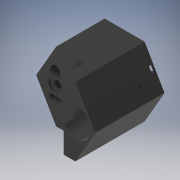
# Autodesk Inventor part: TA02
Saved by Autodesk Inventor 2017 (Build 210142000, 142)
## iProperties
Created: 2018-10-09
Part Number: TA02
Material: ABS Plastic
Document SubType Name: Modeling
Designer: Zach
Density: 1.06 g/cm^3
Appearance: Smooth - Black
Mass: 254.186 g
Surface Area: 673.602 cm^2
Volume: 239.798 cm^3
Author: Zach
Autodesk Inventor part; units mm, degrees
(part 1 of 2)
ref_plane "YZ Plane" through (0, 0, 0) normal (1, 0, 0) x (0, 1, 0)
ref_plane "XZ Plane" through (0, 0, 0) normal (0, 1, 0) x (-1, 0, 0)
ref_plane "XY Plane" through (0, 0, 0) normal (0, 0, 1) x (1, 0, 0)
sketch "Sketch48" plane through (0, 0, 0) normal (0, 0, 1) x (1, 0, 0)
  line L0 (57.5, 0) -> (28.75, -49.7965)
  line L1 (28.75, -49.7965) -> (-28.75, -49.7965)
  line L2 (-28.75, -49.7965) -> (-57.5, 0)
  line L3 (-57.5, 0) -> (-28.75, 49.7965)
  line L4 (-28.75, 49.7965) -> (28.75, 49.7965)
  line L5 (28.75, 49.7965) -> (57.5, 0)
  circle A0 centre (0, 0) radius 7
  circle A1 centre (30, 0) radius 10 construction
  circle A2 centre (-15, 25.9808) radius 5.5
  line L6 (-15, 25.9808) -> (0, 0) construction
  line L7 (0, 0) -> (30, 0) construction
  line L8 (25.6411, -9) -> (34.3589, -9)
  line L9 (25.6411, 9) -> (34.3589, 9)
  arc A3 (25.6411, 9) -> (25.6411, -9) centre (30, 0) ccw
  arc A4 (34.3589, -9) -> (34.3589, 9) centre (30, 0) ccw
  line L10 (21, 9) -> (39, 9) construction
  line L11 (39, 9) -> (39, -9) construction
  line L12 (39, -9) -> (21, -9) construction
  line L13 (21, -9) -> (21, 9) construction
  circle A5 centre (21, 9) radius 2
  circle A6 centre (21, -9) radius 2
  circle A7 centre (39, -9) radius 2
  circle A8 centre (39, 9) radius 2
  point P0 (30, 9)
  point P1 (39, 0)
  dimension "d220" = 115
  dimension "d221" = 14
  dimension "d222" = 30
  dimension "d224" = 30
  dimension "d225" = 120
  dimension "d227" = 11
  dimension "d228" = 20
  dimension "d229" = 18
  dimension "d232" = 18
  dimension "d233" = 18
  dimension "d234" = 4
  dimension "d235" = 4
  dimension "d236" = 4
  dimension "d237" = 4
  constraints: 28 end point, 9 centre point, 8 point on circle, 6 coincident, 3 horizontal, 3 parallel, 2 concentric, 2 horizontal alignment, 2 midpoint, 2 vertical alignment, 1 perpendicular, 13 other
  measures "d220" distance of L0.start L2.end
  measures "d221" diameter of A0
  measures "d222" distance of L7.end point (0, 0)
  measures "d224" distance of point (0, 0) L6.start
  measures "d225" angle of L6 L7
  measures "d227" diameter of A2
  measures "d228" diameter of A1
  measures "d229" distance between parallel lines of L8 L9
  measures "d232" distance of L11.end L12.end
  measures "d233" distance of L10.end L11.end
  measures "d234" diameter of A5
  measures "d235" diameter of A6
  measures "d236" diameter of A7
  measures "d237" diameter of A8
extrude "Extrusion43" add sketch "Sketch48" along normal blind 120
sketch "Sketch49" plane through (0, 0, 0) normal (0, 0, -1) x (-1, 0, 0)
  arc A0 (-34.3589, 9) -> (-34.3589, -9) centre (-30, 0) ccw projected
  circle A1 centre (-30, 0) radius 16.5
  point P0 (0, 0)
  dimension "d238" = 33
  constraints: 1 centre point, 1 coincident
  measures "d238" diameter of A1
extrude "Extrusion44" cut sketch "Sketch49" against normal blind 115
sketch "Sketch50" plane through (0, 0, 0) normal (0, 0, -1) x (-1, 0, 0)
  arc A0 (-34.3589, 9) -> (-34.3589, -9) centre (-30, 0) ccw projected
  circle A1 centre (-30, 0) radius 20
  point P0 (0, 0)
  dimension "d241" = 40
  constraints: 1 centre point, 1 coincident
  measures "d241" diameter of A1
extrude "Extrusion45" cut sketch "Sketch50" against normal blind 75
sketch "Sketch51" plane through (0, 0, 120) normal (0, 0, 1) x (1, 0, 0)
  circle A0 centre (21, 9) radius 2 projected
  arc A1 (25.6411, 9) -> (25.6411, -9) centre (30, 0) ccw projected
  circle A2 centre (21, 9) radius 4.5
  circle A3 centre (21, -9) radius 4.5
  circle A4 centre (39, -9) radius 4.5
  circle A5 centre (39, 9) radius 4.5
  point P0 (0, 0)
  dimension "d244" = 9
  dimension "d247" = 360
  constraints: 4 centre point, 1 coincident, 9 other
  measures "d244" diameter of A2
extrude "Extrusion46" cut sketch "Sketch51" against normal blind 2 contours A0 | A2 A1 | A1 A2 | A3 A1 | A1 A3 | A4 | A5
sketch "Sketch53" plane through (0, 0, 120) normal (0, 0, 1) x (1, 0, 0)
  circle A0 centre (-15, 25.9808) radius 5.5 projected
  circle A1 centre (-15, 25.9808) radius 10
  point P0 (0, 0)
  dimension "d251" = 20
  constraints: 1 centre point, 1 coincident
  measures "d251" diameter of A1
extrude "Extrusion47" cut sketch "Sketch53" against normal blind 5 contours A0 | A1
sketch "Sketch54" plane through (0, 0, 120) normal (0, 0, 1) x (1, 0, 0)
  circle A0 centre (0, 0) radius 12.7
  dimension "d254" = 25.4
  constraints: 1 centre point, 1 coincident
  measures "d254" diameter of A0
extrude "Extrusion48" cut sketch "Sketch54" against normal blind 3.2
sketch "Sketch55" plane through (0, 0, 120) normal (0, 0, 1) x (1, 0, 0)
  circle A0 centre (0, 0) radius 9.56
  dimension "d257" = 19.12
  constraints: 1 centre point, 1 coincident
  measures "d257" diameter of A0
extrude "Extrusion49" cut sketch "Sketch55" against normal blind 12.7
sketch "Sketch56" plane through (0, 0, 0) normal (0, 0, -1) x (-1, 0, 0)
  line L0 (57.5, 0) -> (28.75, 49.7965) projected
  line L1 (28.75, -49.7965) -> (57.5, 0) projected
  line L2 (-28.75, -49.7965) -> (28.75, -49.7965) projected
  line L3 (-57.5, 0) -> (-28.75, -49.7965) projected
  line L4 (-28.75, 49.7965) -> (-57.5, 0) projected
  line L5 (28.75, 49.7965) -> (-28.75, 49.7965) projected
  line L6 (-24.1312, 41.7965) -> (-48.2624, 0)
  line L7 (-48.2624, 0) -> (-24.1312, -41.7965)
  line L8 (-24.1312, -41.7965) -> (24.1312, -41.7965)
  line L9 (24.1312, -41.7965) -> (48.2624, 0)
  line L10 (48.2624, 0) -> (24.1312, 41.7965)
  line L11 (24.1312, 41.7965) -> (-24.1312, 41.7965)
  point P0 (0, 0)
  dimension "d260" = 8
  constraints: 12 end point, 5 other
  measures "d260" distance between parallel lines of L5 L11
extrude "Extrusion50" cut sketch "Sketch56" against normal blind 15 contours L11 L10 L9 L8 L7 L6
sketch "Sketch57" plane through (0, 0, 15) normal (0, 0, -1) x (-1, 0, 0)
  circle A0 centre (0, 0) radius 9.56 projected
extrude "Extrusion51" cut sketch "Sketch57" against normal blind 10
sketch "Sketch58" plane through (0, 0, 0) normal (0, 0, -1) x (-1, 0, 0)
  circle A0 centre (-25.5, -44.1673) radius 2
  circle A1 centre (25.5, -44.1673) radius 2
  circle A2 centre (51, 0) radius 2
  circle A3 centre (25.5, 44.1673) radius 2
  circle A4 centre (-25.5, 44.1673) radius 2
  circle A5 centre (-51, 0) radius 2
  line L0 (-51, 0) -> (51, 0) construction
  point P0 (0, 0)
  point P1 (0, 0)
  dimension "d268" = 360
  dimension "d331" = 102
  dimension "d332" = 4
  constraints: 6 centre point, 2 end point, 1 coincident, 1 horizontal, 1 midpoint, 13 other
  measures "d331" distance of L0.start L0.end
  measures "d332" diameter of A0
extrude "Extrusion52" cut sketch "Sketch58" against normal blind 50
sketch "Sketch59" plane through (0, 0, 0) normal (0, 0, -1) x (-1, 0, 0)
  line L0 (-24.1312, 41.7965) -> (24.1312, 41.7965) construction
  line L1 (28.75, 49.7965) -> (-28.75, 49.7965) construction
  line L2 (0, 41.7965) -> (0, 49.7965) construction
  circle A0 centre (0, 45.7965) radius 2.5
  circle A1 centre (-39.6609, 22.8982) radius 2.5
  circle A2 centre (-39.6609, -22.8982) radius 2.5
  circle A3 centre (0, -45.7965) radius 2.5
  circle A4 centre (39.6609, -22.8982) radius 2.5
  circle A5 centre (39.6609, 22.8982) radius 2.5
  point P0 (0, 0)
  dimension "d272" = 5
  dimension "d275" = 360
  constraints: 6 centre point, 3 midpoint, 2 end point, 13 other
  measures "d272" diameter of A0
extrude "Extrusion53" cut sketch "Sketch59" against normal blind 35
sketch "Sketch60" plane through (0, 0, 15) normal (0, 0, -1) x (-1, 0, 0)
  circle A0 centre (15, 25.9808) radius 5.5 construction
  line L0 (21.5753, 12.3695) -> (-0.0753, 24.8695)
  line L1 (-0.0753, 24.8695) -> (8.4247, 39.592)
  line L2 (8.4247, 39.592) -> (30.0753, 27.092)
  line L3 (30.0753, 27.092) -> (21.5753, 12.3695)
  line L4 (21.5753, 12.3695) -> (8.4247, 39.592) construction
  line L5 (-0.0753, 24.8695) -> (30.0753, 27.092) construction
  line L6 (0, 0) -> (15, 25.9808) construction
  point P0 (10.75, 18.6195)
  dimension "d279" = 17
  dimension "d280" = 25
  constraints: 14 end point, 3 midpoint, 2 parallel, 1 perpendicular, 1 point on line
  measures "d279" distance of L0.end L1.end
  measures "d280" distance of L1.end L2.end
extrude "Extrusion54" cut sketch "Sketch60" against normal blind 94
sketch "Sketch61" plane through (0, 0, 15) normal (0, 0, -1) x (-1, 0, 0)
  line L0 (-7.5897, -33.1458) -> (24.9103, 23.1458)
  line L1 (24.9103, 23.1458) -> (44.8288, 11.6458)
  line L2 (44.8288, 11.6458) -> (12.3288, -44.6458)
  line L3 (12.3288, -44.6458) -> (-7.5897, -33.1458)
  line L4 (-7.5897, -33.1458) -> (44.8288, 11.6458) construction
  line L5 (24.9103, 23.1458) -> (12.3288, -44.6458) construction
  line L6 (18.6195, -10.75) -> (0, 0)
  line L7 (0, 0) -> (0, 4.3773)
  point P0 (8.6603, -5)
  dimension "d283" = 65
  dimension "d284" = 23
  dimension "d285" = 10
  dimension "d286" = 120
  constraints: 16 end point, 3 midpoint, 2 parallel, 1 perpendicular, 1 point on line, 1 vertical
  measures "d283" distance of L1.end L2.end
  measures "d284" distance of L0.end L1.end
  measures "d285" distance from line of L6.end L0
  measures "d286" angle of L7 L6
extrude "Extrusion55" cut sketch "Sketch61" along normal blind 15 and the other way blind 80
sketch "Sketch63" plane through (0, 0, 0) normal (1, 0, 0) x (0, 1, 0)
  line L0 (-41.7965, 15) -> (-41.7965, 0) projected
  line L1 (-41.7965, 0) -> (-41.7965, 15) projected
  line L2 (8.7965, 15) -> (-41.7965, 15) projected
  line L3 (0, 15) -> (-41.7965, 15) projected
  line L4 (8.7965, 15) -> (0, 15) projected
  line L5 (-13.7965, 15) -> (-38.7965, 15)
  line L6 (-38.7965, 15) -> (-38.7965, 0)
  line L7 (-38.7965, 0) -> (-13.7965, 0)
  line L8 (-13.7965, 0) -> (-13.7965, 15)
  point P0 (0, 0)
  dimension "d300" = 25
  dimension "d301" = 15
  dimension "d302" = 3
  constraints: 8 end point, 2 parallel, 1 horizontal, 1 perpendicular, 1 point on line
  measures "d300" distance of L7.end L6.end
  measures "d301" distance of L6.end L5.end
  measures "d302" distance between parallel lines of L1 L6
extrude "Extrusion57" cut sketch "Sketch63" against normal through all
sketch "Sketch66" plane through (0, 0, 120) normal (0, 0, 1) x (1, 0, 0)
  line L0 (-28.75, 49.7965) -> (28.75, 49.7965) projected
  line L1 (10, 49.7965) -> (10, -49.7965)
  line L2 (-28.75, -49.7965) -> (28.75, -49.7965) projected
  line L3 (10, 49.7965) -> (28.75, 49.7965)
  line L4 (10, -49.7965) -> (28.75, -49.7965)
  line L5 (57.5, 0) -> (28.75, 49.7965) projected
  line L6 (28.75, -49.7965) -> (57.5, 0) projected
  point P0 (0, 0)
  dimension "d317" = 10
  constraints: 6 end point, 2 collinear, 2 point on line, 1 vertical
  measures "d317" distance from line of point (0, 0) L1
extrude "Extrusion58" cut sketch "Sketch66" against normal blind 40
sketch "Sketch67" plane through (0, 0, 120) normal (0, 0, 1) x (1, 0, 0)
  line L0 (10, 7.8288) -> (10, 49.7965) projected
  line L1 (10, 49.7965) -> (-28.75, 49.7965) projected
  line L2 (-28.75, 49.7965) -> (-57.5, 0) projected
  line L3 (-57.5, 0) -> (-28.75, -49.7965) projected
  line L4 (-28.75, -49.7965) -> (10, -49.7965) projected
  line L5 (10, -49.7965) -> (10, -7.8288) projected
  arc A0 (10, 7.8288) -> (10, -7.8288) centre (0, 0) ccw projected
  circle A1 centre (-15, 25.9808) radius 10 projected
  line L6 (10, -7.8288) -> (10, 7.8288) projected
extrude "Extrusion59" cut sketch "Sketch67" against normal blind 70 contours A0 L5 L4 L3 L2 L1 L0 | L6 A0 | A1
sketch "Sketch68" plane through (0, 0, 50) normal (0, 0, 1) x (1, 0, 0)
  circle A0 centre (0, 0) radius 8.0625
  dimension "d337" = 16.125
  constraints: 1 centre point, 1 coincident
  measures "d337" diameter of A0
extrude "Extrusion60" cut sketch "Sketch68" against normal blind 13.7
sketch "Sketch69" plane through (10, -49.7965, 80) normal (-1, 0, 0) x (0, 0, 1)
  line L0 (0, 0) -> (-30, 0) projected
  line L1 (-30, 99.5929) -> (0, 99.5929) projected
  circle A0 centre (-15, 24.8982) radius 10
  line L2 (0, 49.7965) -> (0, 0) projected
  line L3 (0, 49.7965) -> (0, 0)
  line L4 (0, 49.7965) -> (0, 99.5929)
  line L5 (-15, 14.8982) -> (-80, 14.8982)
  line L6 (-80, 14.8982) -> (-80, 34.8982)
  line L7 (-80, 34.8982) -> (-15, 34.8982)
  line L8 (-80, 0) -> (-80, 49.7965) projected
  line L9 (0, 49.7965) -> (-80, 49.7965)
  circle A1 centre (-15, 74.6947) radius 10
  line L10 (-15, 84.6947) -> (-80, 84.6947)
  line L11 (-80, 84.6947) -> (-80, 64.6947)
  line L12 (-80, 64.6947) -> (-15, 64.6947)
  point P0 (-15, 0)
  point P1 (0, 24.8982)
  dimension "d324" = 20
  constraints: 18 end point, 5 symmetric about line, 4 point on circle, 2 centre point, 2 midpoint, 2 perpendicular, 2 tangent, 2 vertical, 2 vertical alignment, 1 horizontal, 1 horizontal alignment, 1 point on line, 1 other
  measures "d324" diameter of A0
extrude "Extrusion61" cut sketch "Sketch69" along normal mid plane 5
sketch "Sketch70" plane through (0, 0, 50) normal (0, 0, 1) x (1, 0, 0)
  circle A0 centre (0, 0) radius 9.56 projected
  line L0 (0, -9.56) -> (30, -9.56)
  line L1 (30, -9.56) -> (30, 9.56)
  line L2 (30, 9.56) -> (0, 9.56)
  arc A1 (0, 9.56) -> (0, -9.56) centre (0, 0) ccw
  arc A2 (37.5759, 18.5096) -> (37.5759, -18.5096) centre (30, 0) ccw projected
  constraints: 6 end point, 4 point on circle, 4 tangent, 1 centre point, 1 horizontal, 1 horizontal alignment, 1 midpoint, 1 perpendicular
extrude "Extrusion62" cut sketch "Sketch70" along normal through all
sketch "Sketch71" plane through (10, 49.7965, 50) normal (-1, 0, 0) x (0, 0, 1)
  line L0 (0, -40.2365) -> (30, -40.2365) projected
  line L1 (30, -40.2365) -> (30, 0) projected
  line L2 (0, 0) -> (30, 0) projected
  line L3 (0, 0) -> (0, -14.8982) projected
  line L4 (0, -14.8982) -> (15, -14.8982) projected
  arc A0 (15, -34.8982) -> (15, -14.8982) centre (15, -24.8982) ccw projected
  line L5 (15, -34.8982) -> (0, -34.8982) projected
  line L6 (0, -34.8982) -> (0, -40.2365) projected
  line L7 (30, -59.3565) -> (0, -59.3565) projected
  line L8 (0, -59.3565) -> (0, -64.6947) projected
  line L9 (0, -64.6947) -> (15, -64.6947) projected
  arc A1 (15, -84.6947) -> (15, -64.6947) centre (15, -74.6947) ccw projected
  line L10 (15, -84.6947) -> (0, -84.6947) projected
  line L11 (0, -84.6947) -> (0, -99.5929) projected
  line L12 (30, -99.5929) -> (0, -99.5929) projected
  line L13 (30, -99.5929) -> (30, -59.3565) projected
  point P0 (-50, -49.7965)
extrude "Extrusion63" cut sketch "Sketch71" against normal blind 1
sketch "Sketch72" plane through (0, 0, 15) normal (0, 0, -1) x (-1, 0, 0)
  line L0 (24.1312, 41.7965) -> (39.8936, 14.4952) projected
  line L1 (8.4247, 39.592) -> (30.0753, 27.092) projected
  line L2 (39.8936, 14.4952) -> (30.0753, 27.092)
  line L3 (30.0753, 27.092) -> (27.0753, 21.8958) projected
  line L4 (27.0753, 21.8958) -> (39.8936, 14.4952) projected
  line L5 (30.0753, 27.092) -> (33.8936, 24.8875)
  line L6 (39.8936, 14.4952) -> (33.8936, 24.8875)
  point P0 (0, 0)
  constraints: 6 end point, 2 collinear, 1 point on line
extrude "Extrusion64" cut sketch "Sketch72" against normal through all
sketch "Sketch73" plane through (0, 0, 15) normal (0, 0, -1) x (-1, 0, 0)
  line L0 (-16.5517, 9.56) -> (-12.4328, 9.56) projected
  arc A0 (-12.4328, 9.56) -> (-12.4328, -9.56) centre (-30, 0) ccw projected
  line L1 (-12.4328, -9.56) -> (-16.5517, -9.56) projected
  arc A1 (-16.5517, 9.56) -> (-16.5517, -9.56) centre (-30, 0) ccw projected
  point P0 (0, 0)
extrude "Extrusion65" cut sketch "Sketch73" along normal through all both and the other way through all
sketch "Sketch74" plane through (0, 0, 50) normal (0, 0, 1) x (1, 0, 0)
  line L0 (7.5, -14.8982) -> (7.5, -34.8982) projected
  line L1 (7.5, -14.8982) -> (4.5, -14.8982)
  line L2 (4.5, -14.8982) -> (4.5, -34.8982)
  line L3 (4.5, -34.8982) -> (7.5, -34.8982)
  line L4 (7.5, -34.8982) -> (7.5, -14.8982)
  point P0 (0, 0)
  point P1 (7.5, -32.9904)
  dimension "d338" = 3
  constraints: 8 end point, 2 parallel, 1 coincident, 1 horizontal, 1 perpendicular
  measures "d338" distance of L2.end L0.end
extrude "Extrusion66" add sketch "Sketch74" against normal blind 35
sketch "Sketch75" plane through (12.5, -49.7965, 80) normal (-1, 0, 0) x (0, 0, 1)
  arc A0 (-15, 64.6947) -> (-15, 84.6947) centre (-15, 74.6947) ccw projected
  arc A1 (-15, 14.8982) -> (-15, 34.8982) centre (-15, 24.8982) ccw projected
  circle A2 centre (-15, 74.6947) radius 4
  circle A3 centre (-15, 24.8982) radius 4
  point P0 (-80, 49.7965)
  dimension "d341" = 8
  dimension "d342" = 8
  constraints: 2 centre point, 2 coincident
  measures "d341" diameter of A2
  measures "d342" diameter of A3
extrude "Extrusion67" add sketch "Sketch75" along normal blind 1
fillet "Fillet1" radius 1 2 edges at (11.5, 24.8982, 61) (11.5, -24.8982, 61)
sketch "Sketch76" plane through (0, 0, 15) normal (0, 0, -1) x (-1, 0, 0)
  line L0 (16.9103, 9.2894) -> (3.9199, 16.7894)
  line L1 (3.9199, 16.7894) -> (6.4199, 21.1195)
  line L2 (19.4103, 13.6195) -> (-0.0753, 24.8695) projected
  line L3 (6.4199, 21.1195) -> (19.4103, 13.6195)
  line L4 (19.4103, 13.6195) -> (16.9103, 9.2894)
  line L5 (19.4103, 13.6195) -> (-0.0753, 24.8695) projected
  line L6 (-4.5, -27.7942) -> (19.4103, 13.6195) projected
  point P0 (0, 0)
  dimension "d346" = 15
  dimension "d349" = 5
  constraints: 8 end point, 3 perpendicular, 2 point on line
  measures "d346" distance of L0.start L0.end
  measures "d349" distance of L0.end L1.end
extrude "Extrusion68" cut sketch "Sketch76" against normal through all
sketch "Sketch78" plane through (0, 0, 80) normal (0, 0, 1) x (1, 0, 0)
  circle A0 centre (21.6375, 42.2965) radius 2.5
  line L0 (11, 49.7965) -> (28.75, 49.7965) projected
  point P0 (0, 0)
  dimension "d352" = 21.6375
  dimension "d353" = 7.5
  dimension "d354" = 5
  constraints: 1 centre point
  measures "d352" horizontal distance of point (0, 0) A0.centre
  measures "d353" distance from line of L0 A0.centre
  measures "d354" diameter of A0
extrude "Extrusion69" cut sketch "Sketch78" against normal through all
sketch "Sketch79" plane through (0, 0, 50) normal (0, 0, 1) x (1, 0, 0)
  circle A0 centre (21.6375, 42.2965) radius 2.5 projected
  circle A1 centre (21.6375, 42.2965) radius 10
  line L0 (21.6375, 32.2965) -> (0, 32.2965)
  line L1 (0, 32.2965) -> (0, 52.2965)
  line L2 (0, 52.2965) -> (21.6375, 52.2965)
  point P0 (0, 0)
  dimension "d357" = 20
  constraints: 6 end point, 2 horizontal, 2 point on circle, 2 tangent, 1 centre point, 1 coincident, 1 vertical, 1 vertical alignment
  measures "d357" diameter of A1
extrude "Extrusion70" cut sketch "Sketch79" along normal blind 20 contours A0 | A1 | A1 L0 L1 L2
sketch "Sketch80" plane through (0, 0, 50) normal (0, 0, 1) x (1, 0, 0)
  line L0 (11, 49.7965) -> (11, 9.56) projected
  arc A0 (23.5117, 43.9509) -> (24.0976, 42.7414) centre (21.6375, 42.2965) ccw projected
  line L1 (-6.4199, 21.1195) -> (0.0753, 24.8695) projected
  line L2 (-6.4199, 21.1195) -> (-3.9199, 16.7894) projected
  line L3 (-3.9199, 16.7894) -> (-16.9103, 9.2894) projected
  line L4 (4.5, -27.7942) -> (-16.9103, 9.2894) projected
  line L5 (4.5, -27.7942) -> (4.5, -34.8982) projected
  line L6 (4.5, -34.8982) -> (4.5545, -34.8982) projected
  line L7 (-12.3288, -44.6458) -> (4.5545, -34.8982) projected
  line L8 (-44.8288, 11.6458) -> (-12.3288, -44.6458) projected
  line L9 (-39.8936, 14.4952) -> (-44.8288, 11.6458) projected
  line L10 (-39.8936, 14.4952) -> (-33.8936, 24.8875) projected
  line L11 (-33.8936, 24.8875) -> (-8.4247, 39.592) projected
  line L12 (0.0753, 24.8695) -> (-8.4247, 39.592) projected
  circle A1 centre (0, 0) radius 8.0625 projected
  circle A2 centre (-51, 0) radius 2 projected
  circle A3 centre (-25.5, -44.1673) radius 2 projected
  circle A4 centre (-25.5, 44.1673) radius 2 projected
  line L13 (7.5, 14.8982) -> (7.5, 34.8982) projected
  line L14 (12.5, 34.8982) -> (7.5, 34.8982) projected
  line L15 (12.5, 32.2965) -> (12.5, 34.8982) projected
  line L16 (12.5, 32.2965) -> (21.6375, 32.2965) projected
  arc A5 (21.6375, 32.2965) -> (30.8902, 46.0895) centre (21.6375, 42.2965) ccw projected
  arc A6 (24.0976, 42.7414) -> (23.5117, 43.9509) centre (25.5, 44.1673) ccw projected
  line L17 (-28.75, 49.7965) -> (28.2519, 49.7965) projected
  line L18 (-57.5, 0) -> (-28.75, 49.7965) projected
  line L19 (-28.75, -49.7965) -> (-57.5, 0) projected
  line L20 (11, -49.7965) -> (-28.75, -49.7965) projected
  line L21 (11, -49.7965) -> (11, -34.8982) projected
  line L22 (11, -34.8982) -> (7.5, -34.8982) projected
  line L23 (7.5, -34.8982) -> (7.5, -14.8982) projected
  line L24 (11, -14.8982) -> (7.5, -14.8982) projected
  line L25 (11, -14.8982) -> (11, -9.56) projected
  line L26 (11, -9.56) -> (12.4328, -9.56) projected
  arc A7 (12.4328, 9.56) -> (12.4328, -9.56) centre (30, 0) ccw projected
  line L27 (12.4328, 9.56) -> (11, 9.56) projected
  line L28 (11, 9.56) -> (11, 14.8982) projected
  line L29 (11, 14.8982) -> (7.5, 14.8982) projected
  line L30 (12.5, 32.2965) -> (11, 32.2965)
  line L31 (11, 32.2965) -> (11, 14.8982)
  line L32 (11, 14.8982) -> (12.5, 14.8982)
  line L33 (12.5, 14.8982) -> (12.5, 32.2965)
  line L34 (29.5487, 48.4131) -> (30.8902, 46.0895) projected
  arc A8 (29.5487, 48.4131) -> (28.2519, 49.7965) centre (21.6375, 42.2965) ccw projected
  constraints: 8 end point, 2 parallel, 1 horizontal, 1 perpendicular
extrude "Extrusion71" add sketch "Sketch80" along normal blind 30 contours L30 L33 L32 L0
sketch "Sketch81" plane through (12.5, -49.7965, 80) normal (-1, 0, 0) x (0, 0, 1)
  line L0 (-10, 82.0929) -> (-8.272, 82.0929) projected
  arc A0 (-8.272, 82.0929) -> (-10, 83.3549) centre (-15, 74.6947) ccw projected
  line L1 (-10, 83.3549) -> (-10, 82.0929) projected
  point P0 (-80, 49.7965)
extrude "Extrusion72" add sketch "Sketch81" along normal blind 1.5
sketch "Sketch82" plane through (0, 0, 50) normal (0, 0, 1) x (1, 0, 0)
  line L0 (7.5, 14.8982) -> (7.5, 34.8982) projected
  line L1 (12.5, 34.8982) -> (7.5, 34.8982) projected
  line L2 (7.5, 34.8982) -> (12.5, 34.8982)
  line L3 (12.5, 34.8982) -> (12.5, 14.8982)
  line L4 (12.5, 14.8982) -> (7.5, 14.8982)
  line L5 (7.5, 14.8982) -> (7.5, 34.8982)
  line L6 (7.5, 14.8982) -> (12.5, 14.8982) projected
  line L7 (12.5, 14.8982) -> (12.5, 34.8982) projected
  point P0 (0, 0)
  constraints: 8 end point, 2 parallel, 1 horizontal, 1 perpendicular
extrude "Extrusion73" add sketch "Sketch82" against normal blind 35
sketch "Sketch83" plane through (0, 0, 50) normal (0, 0, 1) x (1, 0, 0)
  line L0 (21.6375, 32.2965) -> (11, 32.2965) projected
  arc A0 (21.6375, 32.2965) -> (30.8902, 46.0895) centre (21.6375, 42.2965) ccw projected
  arc A1 (24.0976, 42.7414) -> (23.5117, 43.9509) centre (25.5, 44.1673) ccw projected
  line L1 (-28.75, 49.7965) -> (28.2519, 49.7965) projected
  line L2 (-57.5, 0) -> (-28.75, 49.7965) projected
  line L3 (-28.75, -49.7965) -> (-57.5, 0) projected
  line L4 (11, -49.7965) -> (-28.75, -49.7965) projected
  line L5 (11, -49.7965) -> (11, -34.8982) projected
  line L6 (11, -34.8982) -> (7.5, -34.8982) projected
  line L7 (7.5, -34.8982) -> (7.5, -14.8982) projected
  line L8 (11, -14.8982) -> (7.5, -14.8982) projected
  line L9 (11, -14.8982) -> (11, -9.56) projected
  line L10 (11, -9.56) -> (12.4328, -9.56) projected
  arc A2 (12.4328, 9.56) -> (12.4328, -9.56) centre (30, 0) ccw projected
  line L11 (12.4328, 9.56) -> (11, 9.56) projected
  line L12 (11, 32.2965) -> (11, 9.56) projected
  arc A3 (23.5117, 43.9509) -> (24.0976, 42.7414) centre (21.6375, 42.2965) ccw projected
  line L13 (-6.4199, 21.1195) -> (0.0753, 24.8695) projected
  line L14 (-6.4199, 21.1195) -> (-3.9199, 16.7894) projected
  line L15 (-3.9199, 16.7894) -> (-16.9103, 9.2894) projected
  line L16 (4.5, -27.7942) -> (-16.9103, 9.2894) projected
  line L17 (4.5, -27.7942) -> (4.5, -34.8982) projected
  line L18 (4.5, -34.8982) -> (4.5545, -34.8982) projected
  line L19 (-12.3288, -44.6458) -> (4.5545, -34.8982) projected
  line L20 (-44.8288, 11.6458) -> (-12.3288, -44.6458) projected
  line L21 (-39.8936, 14.4952) -> (-44.8288, 11.6458) projected
  line L22 (-39.8936, 14.4952) -> (-33.8936, 24.8875) projected
  line L23 (-33.8936, 24.8875) -> (-8.4247, 39.592) projected
  line L24 (0.0753, 24.8695) -> (-8.4247, 39.592) projected
  circle A4 centre (0, 0) radius 8.0625 projected
  circle A5 centre (-51, 0) radius 2 projected
  circle A6 centre (-25.5, -44.1673) radius 2 projected
  circle A7 centre (-25.5, 44.1673) radius 2 projected
  line L25 (11, 49.7965) -> (11, 9.56) projected
  line L26 (11, 9.56) -> (12.4328, 9.56) projected
  arc A8 (12.4328, -9.56) -> (12.4328, 9.56) centre (30, 0) ccw projected
  line L27 (12.4328, -9.56) -> (11, -9.56) projected
  line L28 (11, -9.56) -> (11, -49.7965) projected
  line L29 (28.75, -49.7965) -> (11, -49.7965) projected
  line L30 (57.5, 0) -> (28.75, -49.7965) projected
  line L31 (28.75, 49.7965) -> (57.5, 0) projected
  line L32 (11, 49.7965) -> (28.75, 49.7965) projected
  circle A9 centre (21.6375, 42.2965) radius 2.5 projected
  line L33 (7.5, -14.8982) -> (7.5, -34.8982) projected
  line L34 (12.5, -34.8982) -> (12.5, -14.8982) projected
  line L35 (7.5, -14.8982) -> (12.5, -14.8982)
  line L36 (12.5, -14.8982) -> (12.5, -34.8982)
  line L37 (12.5, -34.8982) -> (7.5, -34.8982)
  line L38 (7.5, -34.8982) -> (7.5, -14.8982)
  line L39 (29.5487, 48.4131) -> (30.8902, 46.0895) projected
  arc A10 (29.5487, 48.4131) -> (28.2519, 49.7965) centre (21.6375, 42.2965) ccw projected
  constraints: 8 end point, 2 parallel, 1 horizontal, 1 perpendicular
extrude "Extrusion74" add sketch "Sketch83" along normal blind 30 and the other way blind 35 contours L6 L7 L8 L28 | L28 L35 L34 L37
sketch "Sketch84" plane through (0, 0, 80) normal (0, 0, 1) x (1, 0, 0)
  circle A0 centre (21.6375, 42.2965) radius 2.5 projected
  line L0 (0, 0) -> (95.1346, 0)
  circle A1 centre (21.6375, -42.2965) radius 2.5
  constraints: 2 end point, 1 centre point, 1 horizontal, 1 symmetric about line, 1 other
extrude "Extrusion75" cut sketch "Sketch84" against normal through all contours A1
sketch "Sketch85" plane through (0, 0, 50) normal (0, 0, 1) x (1, 0, 0)
  line L0 (11, 49.7965) -> (11, 32.2965) projected
  arc A0 (29.5487, 48.4131) -> (28.2519, 49.7965) centre (21.6375, 42.2965) ccw projected
  line L1 (11, 32.2965) -> (21.6375, 32.2965) projected
  circle A1 centre (21.6375, 42.2965) radius 2.5 projected
  line L2 (0, 0) -> (73.6036, 0)
  line L3 (11, -52.2965) -> (11, -32.2965)
  line L4 (21.6375, -52.2965) -> (11, -52.2965)
  arc A2 (21.6375, -52.2965) -> (21.6375, -32.2965) centre (21.6375, -42.2965) ccw
  line L5 (11, -32.2965) -> (21.6375, -32.2965)
  circle A3 centre (21.6375, -42.2965) radius 2.5
  line L6 (30.8902, 46.0895) -> (29.5487, 48.4131) projected
  line L7 (28.2519, 49.7965) -> (11, 49.7965) projected
  arc A4 (21.6375, 32.2965) -> (30.8902, 46.0895) centre (21.6375, 42.2965) ccw projected
  constraints: 8 end point, 4 symmetric about line, 2 centre point, 2 point on circle, 1 horizontal, 2 other
extrude "Extrusion76" cut sketch "Sketch85" along normal blind 20 contours L3 L5 A2 L4
sketch "Sketch86" plane through (0, 0, 50) normal (0, 0, 1) x (1, 0, 0)
  line L0 (11, -9.56) -> (11, -14.8982) projected
  line L1 (7.5, -34.8982) -> (7.5, -14.8982) projected
  line L2 (11, -14.8982) -> (7.5, -14.8982)
  line L3 (7.5, -14.8982) -> (7.5, -34.8982)
  line L4 (7.5, -34.8982) -> (11, -34.8982)
  line L5 (11, -34.8982) -> (11, -14.8982)
  point P0 (0, 0)
  constraints: 8 end point, 2 parallel, 1 horizontal, 1 perpendicular
extrude "Extrusion77" cut sketch "Sketch86" along normal through all
ref_plane "Work Plane2" through (0, 0, 38) normal (0, 0, 1) x (1, 0, 0)
sketch "Sketch87" plane through (0, 0, 38) normal (0, 0, 1) x (1, 0, 0)
  circle A0 centre (21.6375, 42.2965) radius 2.5 projected
  circle A1 centre (21.6375, 42.2965) radius 6.5
  circle A2 centre (21.6375, -42.2965) radius 6.5
  circle A3 centre (21.6375, -42.2965) radius 2.5 projected
  point P0 (0, 0)
  dimension "d377" = 13
  dimension "d378" = 13
  constraints: 2 centre point, 2 coincident
  measures "d377" diameter of A1
  measures "d378" diameter of A2
extrude "Extrusion78" cut sketch "Sketch87" against normal through all
sketch "Sketch88" plane through (0, 0, 80) normal (0, 0, 1) x (1, 0, 0)
  circle A0 centre (21.6375, 42.2965) radius 2.5 projected
  circle A1 centre (21.6375, 42.2965) radius 6.5
  circle A2 centre (21.6375, -42.2965) radius 6.5 projected
  point P0 (0, 0)
  dimension "d381" = 13
  constraints: 1 centre point, 1 coincident
  measures "d381" diameter of A1
extrude "Extrusion79" cut sketch "Sketch88" against normal blind 5
sketch "Sketch89" plane through (11, 49.7965, 50) normal (-1, 0, 0) x (0, 0, 1)
  line L0 (0, -17.5) -> (0, -40.2365) projected
  line L1 (30, -40.2365) -> (0, -40.2365) projected
  line L2 (30, 0) -> (30, -40.2365) projected
  line L3 (20, 0) -> (30, 0) projected
  line L4 (20, 0) -> (20, -17.5) projected
  line L5 (0, -17.5) -> (20, -17.5) projected
  circle A0 centre (15, -28.8682) radius 5
  point P0 (-50, -49.7965)
  point P1 (0, -28.8682)
  dimension "d384" = 10
  dimension "d387" = 15
  constraints: 1 centre point, 1 horizontal alignment, 1 midpoint
  measures "d384" diameter of A0
  measures "d387" distance from line of L0 A0.centre
extrude "Extrusion80" cut sketch "Sketch89" against normal blind 3 contours A0
sketch "Sketch90" plane through (0, 0, 15) normal (0, 0, -1) x (-1, 0, 0)
  circle A0 centre (0, 0) radius 9.56 projected
  arc A1 (-26.3978, 37.8705) -> (-15.1568, 41.7965) centre (-21.6375, 42.2965) ccw projected
  line L0 (-37.5759, 18.5096) -> (-26.3978, 37.8705) projected
  arc A2 (-37.5759, -18.5096) -> (-37.5759, 18.5096) centre (-30, 0) ccw projected
  line L1 (-26.3978, -37.8705) -> (-37.5759, -18.5096) projected
  arc A3 (-15.1568, -41.7965) -> (-26.3978, -37.8705) centre (-21.6375, -42.2965) ccw projected
  line L2 (7.3936, -41.7965) -> (-15.1568, -41.7965) projected
  line L3 (7.3936, -41.7965) -> (-4.5545, -34.8982) projected
  line L4 (-4.5545, -34.8982) -> (-4.5, -34.8982) projected
  line L5 (-4.5, -34.8982) -> (-4.5, -27.7942) projected
  line L6 (-4.5, -27.7942) -> (16.9103, 9.2894) projected
  line L7 (16.9103, 9.2894) -> (3.9199, 16.7894) projected
  line L8 (3.9199, 16.7894) -> (6.4199, 21.1195) projected
  line L9 (6.4199, 21.1195) -> (-0.0753, 24.8695) projected
  line L10 (-0.0753, 24.8695) -> (8.4247, 39.592) projected
  line L11 (8.4247, 39.592) -> (33.8936, 24.8875) projected
  line L12 (24.1312, 41.7965) -> (33.8936, 24.8875) projected
  line L13 (-15.1568, 41.7965) -> (24.1312, 41.7965) projected
  circle A4 centre (39.6609, -22.8982) radius 2.5 projected
  line L14 (43.1838, 8.7965) -> (13.9739, -41.7965) projected
  line L15 (24.1312, -41.7965) -> (13.9739, -41.7965) projected
  line L16 (25.8632, -38.7965) -> (24.1312, -41.7965) projected
  line L17 (25.8632, -38.7965) -> (35.1009, -38.7965) projected
  line L18 (49.5346, -13.7965) -> (35.1009, -38.7965) projected
  line L19 (40.297, -13.7965) -> (49.5346, -13.7965) projected
  line L20 (48.2624, 0) -> (40.297, -13.7965) projected
  line L21 (43.1838, 8.7965) -> (48.2624, 0) projected
  arc A5 (-15.1568, 41.7965) -> (-26.3978, 37.8705) centre (-21.6375, 42.2965) ccw projected
  line L22 (-37.5759, 18.5096) -> (-26.3978, 37.8705) projected
  line L23 (-15.1568, 41.7965) -> (24.1312, 41.7965) projected
  line L24 (24.1312, 41.7965) -> (39.8936, 14.4952) projected
  line L25 (39.8936, 14.4952) -> (44.8288, 11.6458) projected
  line L26 (44.8288, 11.6458) -> (43.1838, 8.7965) projected
  line L27 (43.1838, 8.7965) -> (48.2624, 0) projected
  line L28 (48.2624, 0) -> (40.297, -13.7965) projected
  line L29 (40.297, -13.7965) -> (49.5346, -13.7965) projected
  line L30 (49.5346, -13.7965) -> (57.5, 0) projected
  line L31 (57.5, 0) -> (28.75, 49.7965) projected
  line L32 (28.75, 49.7965) -> (-28.75, 49.7965) projected
  line L33 (-28.75, 49.7965) -> (-57.5, 0) projected
  line L34 (-57.5, 0) -> (-28.75, -49.7965) projected
  line L35 (-28.75, -49.7965) -> (28.75, -49.7965) projected
  line L36 (28.75, -49.7965) -> (35.1009, -38.7965) projected
  line L37 (35.1009, -38.7965) -> (25.8632, -38.7965) projected
  line L38 (25.8632, -38.7965) -> (24.1312, -41.7965) projected
  line L39 (24.1312, -41.7965) -> (13.9739, -41.7965) projected
  line L40 (13.9739, -41.7965) -> (12.3288, -44.6458) projected
  line L41 (12.3288, -44.6458) -> (7.3936, -41.7965) projected
  line L42 (7.3936, -41.7965) -> (-15.1568, -41.7965) projected
  line L43 (-26.3978, -37.8705) -> (-37.5759, -18.5096) projected
  arc A6 (-26.3978, -37.8705) -> (-15.1568, -41.7965) centre (-21.6375, -42.2965) ccw projected
  arc A7 (-49.9286, -1.6888) -> (-37.5759, -18.5096) centre (-30, 0) ccw projected
  arc A8 (-49.9286, 1.6888) -> (-49.9286, -1.6888) centre (-51, 0) ccw projected
  arc A9 (-37.5759, 18.5096) -> (-49.9286, 1.6888) centre (-30, 0) ccw projected
  circle A10 centre (-39.6609, -22.8982) radius 2.5 projected
  circle A11 centre (0, 45.7965) radius 2.5 projected
  circle A12 centre (-39.6609, 22.8982) radius 2.5 projected
  circle A13 centre (0, -45.7965) radius 2.5 projected
  circle A14 centre (39.6609, 22.8982) radius 2.5 projected
  circle A15 centre (51, 0) radius 2 projected
  circle A16 centre (25.5, -44.1673) radius 2 projected
  circle A17 centre (25.5, 44.1673) radius 2 projected
  line L44 (-0.0753, 24.8695) -> (8.4247, 39.592)
  line L45 (8.4247, 39.592) -> (33.8936, 24.8875)
  line L46 (33.8936, 24.8875) -> (25.3936, 10.1651)
  line L47 (25.3936, 10.1651) -> (-0.0753, 24.8695)
  line L48 (3.9199, 16.7894) -> (16.9103, 9.2894)
  line L49 (16.9103, 9.2894) -> (27.9103, 28.342)
  line L50 (27.9103, 28.342) -> (14.9199, 35.842)
  line L51 (14.9199, 35.842) -> (3.9199, 16.7894)
  line L52 (-4.5, -34.8982) -> (-4.5, -27.7942) projected
  line L53 (-4.5, -34.8982) -> (12.3288, -44.6458)
  line L54 (12.3288, -44.6458) -> (44.894, 11.5767)
  line L55 (44.894, 11.5767) -> (28.0652, 21.3243)
  line L56 (28.0652, 21.3243) -> (-4.5, -34.8982)
  constraints: 24 end point, 6 parallel, 4 perpendicular
extrude "Extrusion81" add sketch "Sketch90" against normal blind 35 contours L46 L55 L56 L47 L49 L11 | L49 L47 L51 L11 | L55 L26 L14 L40 L53 L56 L47 L46 | L46 L47 L56 L55 | L51 L9 L10 L11 | L49 L7 L8 L47 | L55 L54 L21 L26 | L21 L54 L15 L14 | L40 L15 L54
sketch "Sketch91" plane through (0, 0, 15) normal (0, 0, -1) x (-1, 0, 0)
  circle A0 centre (0, 0) radius 9.56 projected
  line L0 (24.1312, -41.7965) -> (13.9739, -41.7965) projected
  line L1 (25.8632, -38.7965) -> (24.1312, -41.7965) projected
  line L2 (25.8632, -38.7965) -> (35.1009, -38.7965) projected
  line L3 (49.5346, -13.7965) -> (35.1009, -38.7965) projected
  line L4 (40.297, -13.7965) -> (49.5346, -13.7965) projected
  line L5 (48.2624, 0) -> (40.297, -13.7965) projected
  line L6 (43.1838, 8.7965) -> (48.2624, 0) projected
  line L7 (44.8152, 11.6223) -> (43.1838, 8.7965) projected
  line L8 (44.8152, 11.6223) -> (30.8913, 19.6873) projected
  line L9 (30.8913, 19.6873) -> (33.8936, 24.8875) projected
  line L10 (24.1312, 41.7965) -> (33.8936, 24.8875) projected
  line L11 (-15.1568, 41.7965) -> (24.1312, 41.7965) projected
  line L12 (-37.5759, 18.5096) -> (-26.3978, 37.8705) projected
  arc A1 (-26.3978, 37.8705) -> (-15.1568, 41.7965) centre (-21.6375, 42.2965) ccw projected
  arc A2 (-37.5759, -18.5096) -> (-37.5759, 18.5096) centre (-30, 0) ccw projected
  line L13 (-26.3978, -37.8705) -> (-37.5759, -18.5096) projected
  arc A3 (-15.1568, -41.7965) -> (-26.3978, -37.8705) centre (-21.6375, -42.2965) ccw projected
  line L14 (7.3936, -41.7965) -> (-15.1568, -41.7965) projected
  line L15 (7.3936, -41.7965) -> (-4.5545, -34.8982) projected
  line L16 (-4.5545, -34.8982) -> (-4.5, -34.8982) projected
  line L17 (-4.5, -34.8982) -> (-4.5, -27.7942) projected
  line L18 (-4.5, -27.7942) -> (19.4103, 13.6195) projected
  line L19 (19.4103, 13.6195) -> (22.5519, 11.8057) projected
  line L20 (22.5519, 11.8057) -> (-4.5, -34.8982) projected
  line L21 (-4.5, -34.8982) -> (12.3288, -44.6458) projected
  line L22 (13.9739, -41.7965) -> (12.3288, -44.6458) projected
  circle A4 centre (39.6609, -22.8982) radius 2.5 projected
  line L23 (44.8288, 11.6458) -> (44.8152, 11.6223) projected
  line L24 (39.8936, 14.4952) -> (44.8288, 11.6458) projected
  line L25 (39.8936, 14.4952) -> (33.8936, 24.8875) projected
  line L26 (33.8936, 24.8875) -> (30.8913, 19.6873) projected
  line L27 (30.8913, 19.6873) -> (44.8152, 11.6223) projected
  circle A5 centre (25.5, 44.1673) radius 2 projected
  circle A6 centre (25.5, -44.1673) radius 2 projected
  circle A7 centre (51, 0) radius 2 projected
  circle A8 centre (0, 0) radius 8.0625 projected
  line L28 (12.3288, -44.6458) -> (-4.5, -34.8982) projected
  line L29 (-4.5, -34.8982) -> (22.5519, 11.8057) projected
  line L30 (22.5519, 11.8057) -> (19.4103, 13.6195) projected
  line L31 (19.4103, 13.6195) -> (-4.5, -27.7942) projected
  line L32 (-4.5, -27.7942) -> (-4.5, -34.8982) projected
  line L33 (-4.5, -34.8982) -> (-4.5545, -34.8982) projected
  line L34 (12.3288, -44.6458) -> (-4.5545, -34.8982) projected
  arc A9 (-24.0976, 42.7414) -> (-23.5117, 43.9509) centre (-21.6375, 42.2965) ccw projected
  line L35 (-21.6375, 32.2965) -> (-11, 32.2965) projected
  arc A10 (-30.8902, 46.0895) -> (-21.6375, 32.2965) centre (-21.6375, 42.2965) ccw projected
  arc A11 (-23.5117, 43.9509) -> (-24.0976, 42.7414) centre (-25.5, 44.1673) ccw projected
  line L36 (28.75, 49.7965) -> (-28.2519, 49.7965) projected
  line L37 (57.5, 0) -> (28.75, 49.7965) projected
  line L38 (28.75, -49.7965) -> (57.5, 0) projected
  line L39 (-28.2519, -49.7965) -> (28.75, -49.7965) projected
  arc A12 (-29.5487, -48.4131) -> (-28.2519, -49.7965) centre (-21.6375, -42.2965) ccw projected
  arc A13 (-24.0976, -42.7414) -> (-23.5117, -43.9509) centre (-25.5, -44.1673) ccw projected
  line L40 (-21.6375, -32.2965) -> (-11, -32.2965) projected
  line L41 (-11, -32.2965) -> (-11, -9.56) projected
  line L42 (-11, -9.56) -> (-12.4328, -9.56) projected
  arc A14 (-12.4328, -9.56) -> (-12.4328, 9.56) centre (-30, 0) ccw projected
  line L43 (-12.4328, 9.56) -> (-11, 9.56) projected
  line L44 (-11, 32.2965) -> (-11, 9.56) projected
  arc A15 (-23.5117, -43.9509) -> (-24.0976, -42.7414) centre (-21.6375, -42.2965) ccw projected
  line L45 (-29.5487, 48.4131) -> (-30.8902, 46.0895) projected
  line L46 (-30.8902, -46.0895) -> (-29.5487, -48.4131) projected
  arc A16 (-28.2519, 49.7965) -> (-29.5487, 48.4131) centre (-21.6375, 42.2965) ccw projected
  arc A17 (-21.6375, -32.2965) -> (-30.8902, -46.0895) centre (-21.6375, -42.2965) ccw projected
extrude "Extrusion82" add sketch "Sketch91" against normal blind 35 contours L17 L18 L19 L20 | L34 L15 L16 L21 | L8 L9 L25 L24 L23
sketch "Sketch92" plane through (0, 0, 15) normal (0, 0, -1) x (-1, 0, 0)
  line L0 (13.9739, -41.7965) -> (12.3288, -44.6458) projected
  line L1 (7.3936, -41.7965) -> (-15.1568, -41.7965) projected
  line L2 (13.9739, -41.7965) -> (7.3936, -41.7965)
  line L3 (12.3288, -44.6458) -> (7.3936, -41.7965) projected
  line L4 (7.3936, -41.7965) -> (12.3288, -44.6458)
  line L5 (24.1312, -41.7965) -> (13.9739, -41.7965) projected
  line L6 (12.3288, -44.6458) -> (13.9739, -41.7965)
  line L7 (43.1838, 8.7965) -> (48.2624, 0) projected
  line L8 (43.1838, 8.7965) -> (39.8936, 14.4952)
  line L9 (39.8936, 14.4952) -> (44.8288, 11.6458) projected
  line L10 (39.8936, 14.4952) -> (44.8288, 11.6458)
  line L11 (44.8288, 11.6458) -> (43.1838, 8.7965) projected
  line L12 (44.8288, 11.6458) -> (43.1838, 8.7965)
  circle A0 centre (0, 0) radius 9.56 projected
  line L13 (24.1312, -41.7965) -> (13.9739, -41.7965) projected
  line L14 (25.8632, -38.7965) -> (24.1312, -41.7965) projected
  line L15 (25.8632, -38.7965) -> (35.1009, -38.7965) projected
  line L16 (49.5346, -13.7965) -> (35.1009, -38.7965) projected
  line L17 (40.297, -13.7965) -> (49.5346, -13.7965) projected
  line L18 (48.2624, 0) -> (40.297, -13.7965) construction
  line L19 (43.1838, 8.7965) -> (48.2624, 0) projected
  line L20 (44.8288, 11.6458) -> (43.1838, 8.7965) projected
  line L21 (39.8936, 14.4952) -> (44.8288, 11.6458) projected
  line L22 (24.1312, 41.7965) -> (39.8936, 14.4952) projected
  line L23 (-15.1568, 41.7965) -> (24.1312, 41.7965) projected
  line L24 (-37.5759, 18.5096) -> (-26.3978, 37.8705) projected
  arc A1 (-26.3978, 37.8705) -> (-15.1568, 41.7965) centre (-21.6375, 42.2965) ccw projected
  arc A2 (-37.5759, -18.5096) -> (-37.5759, 18.5096) centre (-30, 0) ccw projected
  line L25 (-26.3978, -37.8705) -> (-37.5759, -18.5096) projected
  arc A3 (-15.1568, -41.7965) -> (-26.3978, -37.8705) centre (-21.6375, -42.2965) ccw projected
  line L26 (7.3936, -41.7965) -> (-15.1568, -41.7965) projected
  line L27 (12.3288, -44.6458) -> (7.3936, -41.7965) projected
  line L28 (13.9739, -41.7965) -> (12.3288, -44.6458) projected
  circle A4 centre (39.6609, -22.8982) radius 2.5 projected
  point P0 (-24.1312, -41.7965)
  constraints: 12 end point, 4 collinear, 2 perpendicular
extrude "Extrusion83" add sketch "Sketch92" along normal blind 15 contours L0 L3 L2 | L8 L9 L11
sketch "Sketch93" plane through (0, 0, 15) normal (0, 0, -1) x (-1, 0, 0)
  line L0 (38.5, -12.5) -> (21.5, -12.5)
  line L1 (21.5, -12.5) -> (21.5, 12.5)
  line L2 (21.5, 12.5) -> (38.5, 12.5)
  line L3 (38.5, 12.5) -> (38.5, -12.5)
  line L4 (30, -12.5) -> (30, 12.5) construction
  line L5 (38.5, 0) -> (21.5, 0) construction
  point P0 (0, 0)
  point P1 (30, 0)
  dimension "d394" = 17
  dimension "d395" = 25
  dimension "d396" = 30
  constraints: 12 end point, 5 midpoint, 2 parallel, 1 horizontal, 1 horizontal alignment, 1 perpendicular
  measures "d394" distance of L1.end L2.end
  measures "d395" distance of L0.end L1.end
  measures "d396" distance of point (0, 0) point (30, 0)
extrude "Extrusion84" cut sketch "Sketch93" against normal through all
sketch "Sketch94" plane through (14, 20.9282, 65) normal (-1, 0, 0) x (0, 0, 1)
  circle A0 centre (0, 0) radius 5 projected
  point P0 (-65, -20.9282)
extrude "Extrusion85" add sketch "Sketch94" along normal blind 3
sketch "Sketch95" plane through (0, 0, 50) normal (0, 0, 1) x (1, 0, 0)
  circle A0 centre (-30, 0) radius 5.5
  line L0 (-21.5, -12.5) -> (-38.5, -12.5) projected
  line L1 (-38.5, -12.5) -> (-21.5, -12.5) projected
  line L2 (-21.5, -12.5) -> (-38.5, -12.5)
  line L3 (-38.5, -12.5) -> (-38.5, -19.5)
  line L4 (-38.5, -19.5) -> (-21.5, -19.5)
  line L5 (-21.5, -19.5) -> (-21.5, -12.5)
  line L6 (-38.5, -12.5) -> (-38.5, 12.5) projected
  line L7 (-38.5, 12.5) -> (-21.5, 12.5) projected
  line L8 (-21.5, 12.5) -> (-21.5, -12.5) projected
  line L9 (-21.5, -12.5) -> (-38.5, -12.5) projected
  circle A1 centre (-25.5, 44.1673) radius 2 projected
  circle A2 centre (-25.5, -44.1673) radius 2 projected
  circle A3 centre (-51, 0) radius 2 projected
  circle A4 centre (0, 0) radius 8.0625 projected
  arc A5 (23.5117, 43.9509) -> (24.0976, 42.7414) centre (21.6375, 42.2965) ccw projected
  line L10 (21.6375, 32.2965) -> (11, 32.2965) projected
  arc A6 (21.6375, 32.2965) -> (30.8902, 46.0895) centre (21.6375, 42.2965) ccw projected
  arc A7 (24.0976, 42.7414) -> (23.5117, 43.9509) centre (25.5, 44.1673) ccw projected
  line L11 (-28.75, 49.7965) -> (28.2519, 49.7965) projected
  line L12 (-57.5, 0) -> (-28.75, 49.7965) projected
  line L13 (-28.75, -49.7965) -> (-57.5, 0) projected
  line L14 (28.2519, -49.7965) -> (-28.75, -49.7965) projected
  arc A8 (28.2519, -49.7965) -> (29.5487, -48.4131) centre (21.6375, -42.2965) ccw projected
  arc A9 (23.5117, -43.9509) -> (24.0976, -42.7414) centre (25.5, -44.1673) ccw projected
  line L15 (21.6375, -32.2965) -> (11, -32.2965) projected
  line L16 (11, -32.2965) -> (11, -9.56) projected
  line L17 (11, -9.56) -> (12.4328, -9.56) projected
  arc A10 (12.4328, 9.56) -> (12.4328, -9.56) centre (30, 0) ccw projected
  line L18 (12.4328, 9.56) -> (11, 9.56) projected
  line L19 (11, 32.2965) -> (11, 9.56) projected
  arc A11 (24.0976, -42.7414) -> (23.5117, -43.9509) centre (21.6375, -42.2965) ccw projected
  line L20 (29.5487, 48.4131) -> (30.8902, 46.0895) projected
  line L21 (30.8902, -46.0895) -> (29.5487, -48.4131) projected
  arc A12 (29.5487, 48.4131) -> (28.2519, 49.7965) centre (21.6375, 42.2965) ccw projected
  arc A13 (30.8902, -46.0895) -> (21.6375, -32.2965) centre (21.6375, -42.2965) ccw projected
  point P0 (-30, -12.5)
  dimension "d401" = 11
  dimension "d402" = 7
  constraints: 8 end point, 2 parallel, 1 centre point, 1 horizontal, 1 horizontal alignment, 1 midpoint, 1 perpendicular, 1 vertical alignment
  measures "d401" diameter of A0
  measures "d402" distance of L0.end L3.end
extrude "Extrusion86" cut sketch "Sketch95" against normal through all contours L5 L4 L3 L0
extrude "Extrusion87" add sketch "Sketch95" against normal blind 5 contours L0 L6 L7 L8
sketch "Sketch96" plane through (0, 0, 50) normal (0, 0, 1) x (1, 0, 0)
  circle A0 centre (-30, 0) radius 5.5 projected
  circle A1 centre (-30, 0) radius 10
  point P0 (0, 0)
  dimension "d407" = 20
  constraints: 1 centre point, 1 coincident
  measures "d407" diameter of A1
extrude "Extrusion88" cut sketch "Sketch96" against normal blind 3.2
sketch "Sketch97" plane through (0, 0, 15) normal (0, 0, -1) x (-1, 0, 0)
  line L0 (21.5, 12.5) -> (38.5, 12.5) projected
  circle A0 centre (30, 19.5) radius 2.5
  circle A1 centre (30, 19.5) radius 6.5
  line L1 (38.5, 12.5) -> (36.2972, 21.1109)
  line L2 (21.5, 12.5) -> (23.7028, 21.1109)
  point P0 (0, 0)
  point P1 (30, 12.5)
  dimension "d410" = 5
  dimension "d411" = 13
  dimension "d412" = 7
  constraints: 4 end point, 2 centre point, 2 point on circle, 2 tangent, 1 coincident, 1 midpoint, 1 vertical alignment
  measures "d410" diameter of A0
  measures "d411" diameter of A1
  measures "d412" distance from line of L0 A0.centre
extrude "Extrusion89" cut sketch "Sketch97" along normal through all both and the other way through all contours L2 A1 L1 L0 | A1 | A0
sketch "Sketch98" plane through (0, 0, 0) normal (0, 0, -1) x (-1, 0, 0)
  circle A0 centre (25.5, 44.1673) radius 2 projected
  circle A1 centre (25.5, -44.1673) radius 2 projected
  circle A2 centre (51, 0) radius 2 projected
  circle A3 centre (39.6609, 22.8982) radius 2.5 projected
  circle A4 centre (0, -45.7965) radius 2.5 projected
  circle A5 centre (-39.6609, 22.8982) radius 2.5 projected
  circle A6 centre (0, 45.7965) radius 2.5 projected
  circle A7 centre (-39.6609, -22.8982) radius 2.5 projected
  arc A8 (36.2972, 21.1109) -> (34.085, 24.556) centre (30, 19.5) ccw projected
  line L0 (36.2972, 21.1109) -> (36.4748, 20.4167) projected
  line L1 (36.4748, 20.4167) -> (48.2624, 0) projected
  line L2 (48.2624, 0) -> (40.297, -13.7965) projected
  line L3 (40.297, -13.7965) -> (49.5346, -13.7965) projected
  line L4 (49.5346, -13.7965) -> (57.5, 0) projected
  line L5 (57.5, 0) -> (28.75, 49.7965) projected
  line L6 (28.75, 49.7965) -> (-28.75, 49.7965) projected
  line L7 (-28.75, 49.7965) -> (-57.5, 0) projected
  line L8 (-57.5, 0) -> (-28.75, -49.7965) projected
  line L9 (-28.75, -49.7965) -> (28.75, -49.7965) projected
  line L10 (28.75, -49.7965) -> (35.1009, -38.7965) projected
  line L11 (35.1009, -38.7965) -> (25.8632, -38.7965) projected
  line L12 (25.8632, -38.7965) -> (24.1312, -41.7965) projected
  line L13 (24.1312, -41.7965) -> (-15.1568, -41.7965) projected
  line L14 (-26.3978, -37.8705) -> (-37.5759, -18.5096) projected
  arc A9 (-26.3978, -37.8705) -> (-15.1568, -41.7965) centre (-21.6375, -42.2965) ccw projected
  arc A10 (-49.9286, -1.6888) -> (-37.5759, -18.5096) centre (-30, 0) ccw projected
  arc A11 (-49.9286, 1.6888) -> (-49.9286, -1.6888) centre (-51, 0) ccw projected
  arc A12 (-37.5759, 18.5096) -> (-49.9286, 1.6888) centre (-30, 0) ccw projected
  line L15 (-37.5759, 18.5096) -> (-26.3978, 37.8705) projected
  arc A13 (-15.1568, 41.7965) -> (-26.3978, 37.8705) centre (-21.6375, 42.2965) ccw projected
  line L16 (-15.1568, 41.7965) -> (24.1312, 41.7965) projected
  line L17 (24.1312, 41.7965) -> (34.085, 24.556) projected
  line L18 (40.297, -13.7965) -> (25.8632, -38.7965)
  line L19 (35.1009, -38.7965) -> (49.5346, -13.7965)
  line L20 (28.75, -49.7965) -> (57.5, 0) projected
  point P0 (0, 0)
  constraints: 4 end point, 1 collinear
extrude "Extrusion90" add sketch "Sketch98" along normal blind 20 contours A8 L17 L16 A13 L15 A12 A11 A10 L14 A9 L13 L12 L11 L10 L9 L8 L7 L6 L5 L4 L3 L2 L1 L0 | L3 L19 L11 L18
sketch "Sketch100" plane through (0, 0, 15) normal (0, 0, -1) x (-1, 0, 0)
  circle A0 centre (39.6609, -22.8982) radius 2.5 projected
  circle A1 centre (39.6609, -22.8982) radius 2.5 projected
  point P0 (0, 0)
extrude "Extrusion91" add sketch "Sketch100" against normal blind 20
sketch "Sketch101" plane through (0, 0, 50) normal (0, 0, 1) x (1, 0, 0)
  circle A0 centre (21.6375, 42.2965) radius 2.5 projected
  circle A1 centre (21.6375, -42.2965) radius 2.5 projected
  line L0 (11, -32.2965) -> (11, -9.56) projected
  line L1 (11, 32.2965) -> (11, 9.56) projected
  circle A2 centre (21.6375, -42.2965) radius 11.5
  circle A3 centre (21.6375, 42.2965) radius 11.5
  line L2 (21.6375, 53.7965) -> (11, 53.7965)
  line L3 (11, 53.7965) -> (11, 30.7965)
  line L4 (11, 30.7965) -> (21.6375, 30.7965)
  line L5 (21.6375, 30.7965) -> (21.6375, 53.7965)
  line L6 (21.6375, -53.7965) -> (11, -53.7965)
  line L7 (11, -53.7965) -> (11, -30.7965)
  line L8 (11, -30.7965) -> (21.6375, -30.7965)
  line L9 (21.6375, -30.7965) -> (21.6375, -53.7965)
  point P0 (0, 0)
  dimension "d419" = 23
  dimension "d420" = 23
  constraints: 16 end point, 4 parallel, 4 point on circle, 3 coincident, 3 point on line, 2 centre point, 2 horizontal, 2 perpendicular, 1 midpoint
  measures "d419" diameter of A2
  measures "d420" diameter of A3
extrude "Extrusion92" cut sketch "Sketch101" along normal blind 20
sketch "Sketch102" plane through (21.6375, 42.2965, 38) normal (0, 0, -1) x (-1, 0, 0)
  arc A0 (-1.8742, 1.6545) -> (-2.4601, 0.4449) centre (-3.8625, 1.8708) ccw projected
  arc A1 (-2.4601, 0.4449) -> (-1.8742, 1.6545) centre (0, 0) ccw projected
  circle A2 centre (0, 0) radius 6.5 projected
  arc A3 (-2.4601, -85.0378) -> (-1.8742, -86.2474) centre (-3.8625, -86.4638) ccw projected
  arc A4 (-1.8742, -86.2474) -> (-2.4601, -85.0378) centre (0, -84.5929) ccw projected
  circle A5 centre (0, -84.5929) radius 6.5 projected
  point P0 (21.6375, -42.2965)
extrude "Extrusion93" add sketch "Sketch102" along normal blind 58
ref_plane "Work Plane3" through (0, 0, 18.25) normal (0, 0, 1) x (1, 0, 0)
sketch "Sketch103" plane through (0, 0, 18.25) normal (0, 0, 1) x (1, 0, 0)
  arc A0 (23.5117, 43.9509) -> (24.0976, 42.7414) centre (21.6375, 42.2965) ccw projected
  circle A1 centre (21.6375, 42.2965) radius 2.5 projected
  circle A2 centre (21.6375, -42.2965) radius 2.5 projected
  point P0 (0, 0)
extrude "Extrusion94" add sketch "Sketch103" against normal blind 38.25
sketch "Sketch104" plane through (0, 0, 50) normal (0, 0, 1) x (1, 0, 0)
  arc A0 (24.0976, 42.7414) -> (23.5117, 43.9509) centre (25.5, 44.1673) ccw projected
  arc A1 (23.5117, -43.9509) -> (24.0976, -42.7414) centre (25.5, -44.1673) ccw projected
  arc A2 (23.5117, 43.9509) -> (24.0976, 42.7414) centre (21.6375, 42.2965) ccw construction
  arc A3 (24.0976, 42.7414) -> (23.5117, 43.9509) centre (21.6375, 42.2965) ccw projected
  arc A4 (24.0976, -42.7414) -> (23.5117, -43.9509) centre (21.6375, -42.2965) ccw construction
  arc A5 (23.5117, -43.9509) -> (24.0976, -42.7414) centre (21.6375, -42.2965) ccw projected
  arc A6 (24.0976, 42.7414) -> (23.5117, 43.9509) centre (21.6375, 42.2965) ccw
  arc A7 (23.5117, -43.9509) -> (24.0976, -42.7414) centre (21.6375, -42.2965) ccw
  arc A8 (24.0976, 42.7414) -> (23.5117, 43.9509) centre (21.6375, 42.2965) ccw projected
  arc A9 (24.0976, 42.7414) -> (23.5117, 43.9509) centre (25.5, 44.1673) ccw
  arc A10 (24.0976, -42.7414) -> (23.5117, -43.9509) centre (21.6375, -42.2965) ccw projected
  arc A11 (23.5117, -43.9509) -> (23.5117, -43.9509) centre (25.5, -44.1673) ccw
  circle A12 centre (25.5, -44.1673) radius 2
  circle A13 centre (25.5, 44.1673) radius 2
  point P0 (0, 0)
  constraints: 8 point on circle, 5 coincident, 4 centre point, 1 concentric, 6 other
extrude "Extrusion95" add sketch "Sketch104" against normal blind 10 contours A3 A0 | A13 A3 | A5 A1 | A11 A5
sketch "Sketch105" plane through (0, 0, 40) normal (0, 0, -1) x (-1, 0, 0)
  arc A0 (-23.5117, 43.9509) -> (-24.0976, 42.7414) centre (-25.5, 44.1673) ccw projected
  arc A1 (-24.0976, 42.7414) -> (-23.5117, 43.9509) centre (-25.5, 44.1673) ccw projected
  arc A2 (-24.0976, -42.7414) -> (-23.5117, -43.9509) centre (-25.5, -44.1673) ccw projected
  arc A3 (-23.5117, -43.9509) -> (-24.0976, -42.7414) centre (-25.5, -44.1673) ccw projected
  point P0 (0, 0)
extrude "Extrusion96" cut sketch "Sketch105" along normal through all
sketch "Sketch106" plane through (0, 0, 15) normal (0, 0, -1) x (-1, 0, 0)
  line L0 (48.2624, 0) -> (24.1312, -41.7965) projected
  line L1 (24.1312, -41.7965) -> (-24.1312, -41.7965)
  line L2 (-24.1312, -41.7965) -> (-48.2624, 0)
  line L3 (-48.2624, 0) -> (-24.1312, 41.7965)
  line L4 (-24.1312, 41.7965) -> (24.1312, 41.7965)
  line L5 (24.1312, 41.7965) -> (48.2624, 0)
  line L6 (48.2624, 0) -> (24.1312, -41.7965)
  point P0 (0, 0)
  point P1 (0, 0)
  constraints: 12 end point, 1 coincident, 13 other
extrude "Extrusion97" cut sketch "Sketch106" along normal through all
sketch "Sketch107" plane through (0, 0, 50) normal (0, 0, 1) x (1, 0, 0)
  circle A0 centre (-25.5, -44.1673) radius 2 projected
  circle A1 centre (-51, 0) radius 2 projected
  circle A2 centre (-25.5, 44.1673) radius 2 projected
  point P0 (0, 0)